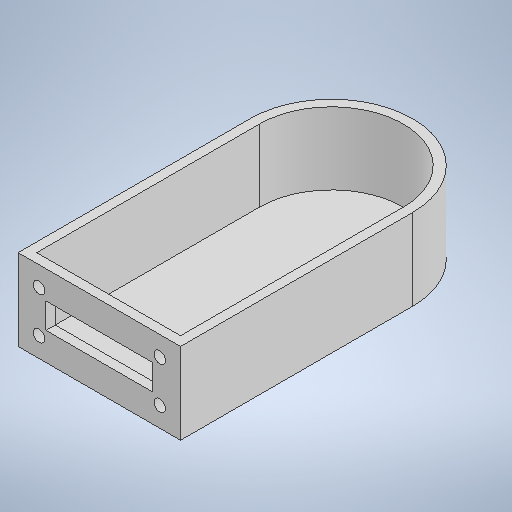
# Autodesk Inventor part: SCARA arm
Saved by Autodesk Inventor 2025.2 (Build 292293000, 293)
## iProperties
Created: 2025-01-27
Part Number: SCARA arm
Material: Generic
Document SubType Name: Modeling
Designer: caomi
Density: 1 g/cm^3
Appearance: Default
Author: caomi
Autodesk Inventor part; units mm, degrees
ref_plane "YZ Plane" through (0, 0, 0) normal (1, 0, 0) x (0, 1, 0)
ref_plane "XZ Plane" through (0, 0, 0) normal (0, 1, 0) x (-1, 0, 0)
ref_plane "XY Plane" through (0, 0, 0) normal (0, 0, 1) x (1, 0, 0)
sketch "Sketch1" plane through (0, 0, 0) normal (0, 1, 0) x (-1, 0, 0)
  line L0 (0, 0) -> (70, 0)
  line L1 (70, 0) -> (70, -100)
  line L2 (70, -100) -> (0, -100)
  line L3 (0, -100) -> (0, 0)
  circle A0 centre (35, -100) radius 35
  point P0 (0, -100)
  dimension "d0" = 70
  dimension "d1" = 100
  constraints: 8 end point, 2 parallel, 1 horizontal, 1 midpoint, 1 perpendicular, 3 other
  measures "d0" distance of L0.start L0.end
  measures "d1" distance between parallel lines of L2 L0
extrude "Extrusion1" add sketch "Sketch1" along normal blind 35
shell "Shell1" thickness 4 removed faces 1 at (-23.3333, 35, -33.3333)
sketch "Sketch2" plane through (-70, 0, 0) normal (0, 0, 1) x (1, 0, 0)
  line L0 (35, 44.7542) -> (35, -30.4775) construction
  line L1 (75.874, 17.5) -> (-5.874, 17.5) construction
  line L2 (0, 35) -> (70, 35) projected
  line L3 (70, 0) -> (70, 35) projected
  line L4 (0, 0) -> (0, 35) projected
  line L5 (0, 0) -> (70, 0) projected
  line L6 (58, 23) -> (12, 23)
  line L7 (12, 23) -> (12, 12)
  line L8 (12, 12) -> (58, 12)
  line L9 (58, 12) -> (58, 23)
  circle A0 centre (9, 26.5) radius 2.5
  circle A1 centre (61, 8.5) radius 2.5
  circle A2 centre (9, 8.5) radius 2.5
  circle A3 centre (61, 26.5) radius 2.5
  point P0 (35, 17.5)
  point P1 (35, 35)
  point P2 (70, 17.5)
  dimension "d7" = 12
  dimension "d8" = 5
  dimension "d9" = 52
  dimension "d10" = 18
  constraints: 12 end point, 4 centre point, 3 midpoint, 3 point on line, 1 equal radius, 1 horizontal, 1 symmetric about line, 1 vertical, 5 other
  measures "d7" distance between parallel lines of L2 L6
  measures "d8" diameter of A1
  measures "d9" distance of A1.centre A2.centre
  measures "d10" distance of A3.centre A1.centre
extrude "Extrusion2" cut sketch "Sketch2" against normal blind 52 contours L9 L8 L7 L6 | A0 | A1 | A2 | A3
equation "\"d11\" = d9"
body "Solid1"
